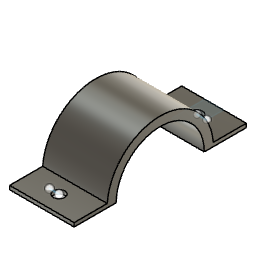
case master entier (Autodesk Fusion 360 archive; units mm, degrees)
design "Piece guidon"
Autodesk Fusion 360 part; units mm, degrees
sketch "Esquisse16" plane through (0, 0, 0) normal (0, 0, 1) x (1, 0, 0)
  line L0 (0, 0) -> (5, 0)
  line L1 (5, 0) -> (5, 25)
  line L2 (5, 25) -> (0, 25)
  line L3 (0, 25) -> (0, 0)
  constraint horizontal L0
  constraint vertical L1
  constraint horizontal L2
  constraint vertical L3
  constraint coincident L0.start L3.end
extrude "Extrusion15" add sketch "Esquisse16" along normal blind 1 makes body 1
extrude "Extrusion16" add 1 faces at (3.3333, 25, 0.3333) along direction (0, 1, 0) blind 50 on bodies 1 bodies 1
extrude "Extrusion17" cut 1 faces at (3.3333, 75, 0.3333) along direction (0, -1, 0) blind 5 on bodies 1 bodies 1
sketch "Esquisse20" plane through (0, 0, 0) normal (-1, 0, 0) x (0, -1, 0)
  line L0 (-70, 1) -> (-70, 0)
  line L1 (-70, 0) -> (0, 0)
  line L2 (0, 0) -> (0, 1)
  line L3 (0, 1) -> (-70, 1)
  arc A0 (-24, 0) -> (-52, 0) centre (-38, 0) ccw
  dimension "d47" = 28
  constraint coincident L1 A0.end
  constraint coincident L1 A0.start
  measures "d47" diameter of A0
extrude "Extrusion21" add sketch "Esquisse20" along normal blind 3 separate body contours L3 A0 makes body 2
extrude "Extrusion22" add 1 faces at (0, 36.5195, 5.8166) along direction (1, 0, 0) blind 5 on bodies 2 bodies 1 2
extrude "Extrusion23" cut 1 faces at (-3, 36.5195, 5.8166) along direction (1, 0, 0) blind 3 on bodies 1 bodies 1
sketch "Esquisse21" plane through (0, 0, 0) normal (1, 0, 0) x (0, 1, 0)
sketch "Esquisse22" plane through (0, 0, 0) normal (-1, 0, 0) x (0, -1, 0)
  line L0 (-70, 1) -> (-70, 0)
  line L1 (-70, 0) -> (0, 0)
  line L2 (0, 0) -> (0, 1)
  line L3 (0, 1) -> (-24.0358, 1)
  arc A0 (-24.0358, 1) -> (-51.9642, 1) centre (-38, 0) ccw
  line L4 (-51.9642, 1) -> (-70, 1)
  arc A1 (-26.4, 0) -> (-49.6, 0) centre (-38, 0) ccw
  dimension "d54" = 23.2
  constraint coincident L1 A1.end
  constraint coincident L1 A1.start
  measures "d54" diameter of A1
extrude "Extrusion24" cut sketch "Esquisse22" against normal blind 13 contours L1 A1 bodies 1
extrude "Extrusion25" cut 1 faces at (1.6667, 0, 0.3333) along direction (0, 1, 0) blind 10 on bodies 1 bodies 1
extrude "Extrusion26" cut 1 faces at (3.3333, 70, 0.3333) along direction (0, -1, 0) blind 10 on bodies 1 bodies 1
extrude "Extrusion27" cut 1 faces at (1.6667, 10, 0.3333) along direction (0, 1, 0) blind 5 on bodies 1 bodies 1
extrude "Extrusion28" cut 1 faces at (1.6667, 15, 0.3333) along direction (0, 1, 0) blind 0.325 on bodies 1 bodies 1
extrude "Extrusion29" add 1 faces at (3.3333, 60, 0.3333) along direction (0, 1, 0) blind 0.675 on bodies 1 bodies 1
sketch "Esquisse23" plane through (0, 0, 1) normal (0, 0, 1) x (-1, 0, 0)
  line L0 (0, -60.675) -> (0, -51.9642)
  line L1 (0, -51.9642) -> (-5, -51.9642)
  line L2 (-5, -51.9642) -> (-5, -60.675)
  line L3 (-5, -60.675) -> (0, -60.675)
  line L4 (0, -19.825) -> (-2.5, -19.825)
  constraint horizontal L4
sketch "Esquisse24" plane through (0, 0, 1) normal (0, 0, 1) x (-1, 0, 0)
  line L0 (0, -15.325) -> (-5, -15.325)
  line L1 (-5, -15.325) -> (-5, -24.0358)
  line L2 (-5, -24.0358) -> (0, -24.0358)
  line L3 (0, -24.0358) -> (0, -15.325)
  circle A0 centre (-2.5, -19.825) radius 1.5
  dimension "d67" = 3
  measures "d67" diameter of A0
extrude "Extrusion30" cut sketch "Esquisse24" against normal blind 4 contours A0 bodies 1
sketch "Esquisse25" plane through (0, 0, 1) normal (0, 0, 1) x (-1, 0, 0)
sketch "Esquisse26" plane through (0, 0, 1) normal (0, 0, 1) x (-1, 0, 0)
  line L0 (-5, -56.175) -> (-2.5, -56.175)
  constraint horizontal L0
sketch "Esquisse27" plane through (0, 0, 1) normal (0, 0, 1) x (-1, 0, 0)
  circle A0 centre (-2.5, -56.175) radius 1.5
  dimension "d70" = 3
  measures "d70" diameter of A0
extrude "Extrusion31" cut sketch "Esquisse27" against normal blind 3 bodies 1
move_face "DécalerLesFaces1" offset 6 1 faces at (0, 37.014, 13.1368) on bodies 1
move_face "DécalerLesFaces2" offset 6 1 faces at (5, 38.986, 13.1368) on bodies 1
sketch "Esquisse19" plane through (0, 0, 0) normal (1, 0, 0) x (0, 1, 0)
  circle A0 centre (35, 0) radius 11.6
  dimension "d40" = 23.2
  measures "d40" diameter of A0
extrude "Extrusion18" [rolled back] along distance -4 taper angle 0
extrude "Extrusion19" [rolled back] along distance 5 taper angle 0
extrude "Extrusion20" [rolled back] along distance -4 taper angle 0
